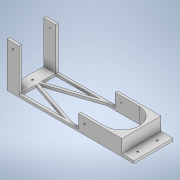
# Autodesk Inventor part: frame
Saved by Autodesk Inventor 2020 (Build 240168000, 168)
## iProperties
Created: 2020-02-29
Part Number: frame
Material: Типовые
Document SubType Name: Modeling
Designer: CSS38
Density: 1 g/cm^3
Appearance: По умолчанию
Author: CSS38
Autodesk Inventor part; units mm, degrees
ref_plane "YZ Plane" through (0, 0, 0) normal (1, 0, 0) x (0, 1, 0)
ref_plane "XZ Plane" through (0, 0, 0) normal (0, 1, 0) x (-1, 0, 0)
ref_plane "XY Plane" through (0, 0, 0) normal (0, 0, 1) x (1, 0, 0)
sketch "Эскиз1" plane through (0, 0, 0) normal (0, 1, 0) x (-1, 0, 0)
  line L0 (-52.75, 16.25) -> (52.75, 16.25)
  line L1 (52.75, 16.25) -> (52.75, -16.25)
  line L2 (52.75, -16.25) -> (-52.75, -16.25)
  line L3 (-52.75, -16.25) -> (-52.75, 16.25)
  line L4 (-52.75, 16.25) -> (52.75, -16.25) construction
  line L5 (52.75, 16.25) -> (-52.75, -16.25) construction
  line L6 (-42.75, -14.25) -> (0, -14.25)
  line L7 (42.75, -14.25) -> (42.75, -2.1082)
  line L8 (42.75, 14.25) -> (6.3246, 14.25)
  line L9 (-42.75, 14.25) -> (-42.75, -14.25)
  line L10 (52.75, -16.25) -> (36.5, 0) construction
  line L11 (36.5, 0) -> (52.75, 16.25) construction
  line L12 (47.75, -16.25) -> (47.75, 16.25) construction
  line L13 (0, -22.75) -> (0, 22.75) construction
  line L14 (0, -16.25) -> (0, -14.25) construction
  line L15 (0, 14.25) -> (0, 16.25) construction
  line L16 (0, -14.25) -> (42.75, 0)
  line L17 (42.75, 0) -> (0, 14.25)
  line L18 (42.75, -2.1082) -> (6.3246, -14.25)
  line L19 (42.75, 2.1082) -> (6.3246, 14.25)
  line L20 (42.75, -2.1082) -> (42.1175, -0.2108) construction
  line L21 (42.75, 2.1082) -> (42.1175, 0.2108) construction
  line L22 (42.75, -2.1082) -> (42.75, 2.1082) construction
  line L23 (42.75, 2.1082) -> (42.75, 14.25)
  line L24 (6.3246, -14.25) -> (42.75, -14.25)
  line L25 (0, -14.25) -> (6.3246, -14.25) construction
  line L26 (6.3246, 14.25) -> (0, 14.25) construction
  line L27 (0, 14.25) -> (-42.75, 14.25)
  point P0 (0, 0)
  point P1 (0, 0)
  dimension "d0" = 105.5
  dimension "d4" = 10
  dimension "d5" = 10
  dimension "d8" = 5
  dimension "d24" = 28.5
  dimension "d29" = 2
  constraints: 54 end point, 16 parallel, 14 perpendicular, 10 point on line, 5 equal length, 4 midpoint, 1 coincident, 1 horizontal
  measures "d0" distance of L1.end L2.end
  measures "d4" distance between parallel lines of L7 L1
  measures "d5" distance between parallel lines of L9 L3
  measures "d8" distance between parallel lines of L1 L12
  measures "d24" distance of L9.start L6.start
  measures "d29" distance of L14.start L6.end
extrude "Выдавливание1" add sketch "Эскиз1" along normal blind 2
sketch "Эскиз2" plane through (0, 0, 0) normal (0, 1, 0) x (-1, 0, 0)
  line L0 (-42.75, -16.25) -> (-42.75, 16.25)
  line L1 (52.75, 16.25) -> (-52.75, 16.25) projected
  line L2 (-52.75, 16.25) -> (-52.75, -16.25) projected
  line L3 (0, -14.25) -> (-42.75, -14.25) construction
  line L4 (-40.75, -14.25) -> (-40.75, 14.25) construction
  line L5 (6.3246, 14.25) -> (42.75, 14.25) construction
  line L6 (-40.75, -14.25) -> (-26.5, -14.25) construction
  line L7 (-6.75, -14.25) -> (-6.75, -16.25)
  line L8 (-52.75, -16.25) -> (52.75, -16.25) projected
  line L9 (-6.75, -16.25) -> (-42.75, -16.25)
  line L10 (-42.75, 16.25) -> (-6.75, 16.25)
  line L11 (-6.75, 14.25) -> (-26.5, 14.25)
  line L12 (-6.75, 14.25) -> (-6.75, 16.25)
  arc A0 (-26.5, 14.25) -> (-26.5, -14.25) centre (-26.5, 0) ccw
  line L13 (-26.5, -14.25) -> (-6.75, -14.25)
  line L14 (-26.5, 14.25) -> (-40.75, 14.25) construction
  line L15 (-42.75, -14.25) -> (-42.75, 14.25) projected
  point P0 (0, 0)
  point P1 (42.75, -14.25)
  point P2 (-42.75, -16.25)
  dimension "d13" = 2
  dimension "d14" = 34
  constraints: 20 end point, 7 point on line, 5 tangent, 4 collinear, 3 perpendicular, 3 vertical, 2 point on circle, 1 centre point
  measures "d13" distance between parallel lines of L0 L4
  measures "d14" distance of L4.start L7.start
extrude "Выдавливание2" add sketch "Эскиз2" along normal blind 13 contours L0 L1 L12 L11 A0 L13 L7 L8
sketch "Эскиз3" plane through (0, 2, 0) normal (0, 1, 0) x (1, 0, 0)
  line L0 (-42.75, 14.25) -> (-52.75, 14.25)
  line L1 (-52.75, 14.25) -> (-52.75, 16.25)
  line L2 (-52.75, 16.25) -> (-42.75, 16.25)
  line L3 (-42.75, 16.25) -> (-42.75, 14.25)
  line L4 (-52.75, 16.25) -> (-52.75, -16.25) construction
  line L5 (-52.75, -16.25) -> (-42.75, -16.25)
  line L6 (-42.75, -16.25) -> (-42.75, -14.25)
  line L7 (-42.75, -14.25) -> (-52.75, -14.25)
  line L8 (-52.75, -14.25) -> (-52.75, -16.25)
  point P0 (0, 0)
  point P1 (-42.75, 14.25)
  constraints: 16 end point, 4 parallel, 2 coincident, 2 horizontal, 2 perpendicular
extrude "Выдавливание3" add sketch "Эскиз3" along normal blind 35
sketch "Эскиз4" plane through (-52.75, 0, 16.25) normal (0, 0, 1) x (1, 0, 0)
  line L0 (10, 37) -> (0, 37) construction
  line L1 (0, 37) -> (10, 37) construction
  line L2 (10, 37) -> (10, 27) construction
  line L3 (10, 27) -> (0, 27) construction
  line L4 (0, 27) -> (0, 37) construction
  line L5 (105.5, 0) -> (0, 0) construction
  line L6 (0, 0) -> (0, 37) construction
  line L7 (10, 37) -> (10, 2) construction
  line L8 (10, 2) -> (59.5, 2) construction
  line L9 (59.5, 2) -> (59.5, 13) construction
  line L10 (59.5, 13) -> (95.5, 13) construction
  line L11 (95.5, 13) -> (95.5, 2) construction
  line L12 (95.5, 2) -> (105.5, 2) construction
  line L13 (105.5, 2) -> (105.5, 0) construction
  line L14 (10, 2) -> (10, 37) construction
  line L15 (0, 0) -> (0, 37) construction
  line L16 (10, 27) -> (0, 37) construction
  line L17 (10, 37) -> (0, 27) construction
  circle A0 centre (5, 32) radius 0.5
  line L18 (59.5, 13) -> (69.5, 13) construction
  line L19 (69.5, 13) -> (69.5, 3) construction
  line L20 (69.5, 3) -> (59.5, 3) construction
  line L21 (59.5, 3) -> (59.5, 13) construction
  line L22 (69.5, 13) -> (59.5, 3) construction
  line L23 (59.5, 2) -> (59.5, 13) construction
  line L24 (59.5, 13) -> (69.5, 3) construction
  circle A1 centre (64.5, 8) radius 0.5
  line L25 (0, 37) -> (10, 37) projected
  point P0 (52.75, 0)
  dimension "d19" = 1
  dimension "d20" = 10
  dimension "d21" = 1
  constraints: 24 end point, 5 perpendicular, 4 parallel, 2 centre point, 2 horizontal, 2 midpoint, 1 collinear
  measures "d19" diameter of A0
  measures "d20" distance of L19.end L20.end
  measures "d21" diameter of A1
hole "Отверстие1" at (-47.75, 32, 16.25) at (11.75, 8, 16.25) direction (0, 0, -1) diameter 1 depth 16.25 countersink diameter 1.5 countersink angle 90
mirror "Зеркальное отражение1" about plane through (0, 0, 0) normal (0, 0, 1) of "Отверстие1"
sketch "Эскиз5" plane through (0, 2, 0) normal (0, 1, 0) x (1, 0, 0)
  line L0 (-42.75, 2.1082) -> (-6.3246, 14.25) construction
  line L1 (-6.3246, 14.25) -> (-42.75, 14.25) construction
  line L2 (-42.75, 14.25) -> (-52.75, 14.25) construction
  line L3 (-52.75, -14.25) -> (-52.75, 14.25) construction
  line L4 (-52.75, -16.25) -> (-52.75, -14.25) construction
  line L5 (-42.75, -16.25) -> (-52.75, -16.25) construction
  line L6 (-42.75, -14.25) -> (-42.75, -16.25) construction
  line L7 (-42.75, -14.25) -> (-6.3246, -14.25) construction
  line L8 (-6.3246, -14.25) -> (-42.75, -2.1082) construction
  line L9 (-42.75, -2.1082) -> (-42.75, -14.25) construction
  line L10 (-42.75, 14.25) -> (-42.75, 2.1082) construction
  line L11 (-42.75, 16.25) -> (-42.75, 14.25) construction
  line L12 (-42.75, 16.25) -> (6.75, 16.25) construction
  line L13 (6.75, 16.25) -> (42.75, 16.25) construction
  line L14 (42.75, 16.25) -> (52.75, 16.25) construction
  line L15 (52.75, 16.25) -> (52.75, -16.25) construction
  line L16 (52.75, -16.25) -> (42.75, -16.25) construction
  line L17 (42.75, 16.25) -> (42.75, -16.25) construction
  line L18 (-52.75, 14.25) -> (-52.75, 16.25) construction
  line L19 (-52.75, 16.25) -> (-42.75, 16.25) construction
  line L20 (-52.75, -14.25) -> (-42.75, -14.25) construction
  line L21 (6.75, -16.25) -> (-42.75, -16.25) construction
  line L22 (42.75, -16.25) -> (6.75, -16.25) construction
  line L23 (6.75, 14.25) -> (6.75, 16.25) construction
  line L24 (6.75, 14.25) -> (0, 14.25) construction
  line L25 (0, 14.25) -> (-42.75, 0) construction
  line L26 (-42.75, 0) -> (0, -14.25) construction
  line L27 (0, -14.25) -> (6.75, -14.25) construction
  line L28 (6.75, -14.25) -> (26.5, -14.25) construction
  arc A0 (26.5, -14.25) -> (26.5, 14.25) centre (26.5, 0) ccw construction
  line L29 (26.5, 14.25) -> (6.75, 14.25) construction
  line L30 (6.75, -16.25) -> (6.75, -14.25) construction
  line L31 (-6.3246, -14.25) -> (-42.75, -14.25) construction
  line L32 (-52.75, 14.25) -> (-42.75, -14.25) construction
  line L33 (-42.75, 14.25) -> (-52.75, -14.25) construction
  line L34 (42.75, 16.25) -> (52.75, 0) construction
  line L35 (52.75, -16.25) -> (52.75, 16.25) construction
  line L36 (52.75, 0) -> (42.75, -16.25) construction
  line L37 (-52.75, -16.25) -> (52.75, -16.25) construction
  line L38 (52.75, -16.25) -> (42.75, 0) construction
  line L39 (52.75, 16.25) -> (-52.75, 16.25) construction
  line L40 (42.75, 0) -> (52.75, 16.25) construction
  circle A1 centre (-47.75, 0) radius 0.5
  circle A2 centre (47.75, 8.125) radius 0.5
  circle A3 centre (47.75, -8.125) radius 0.5
  point P0 (0, 0)
  dimension "d37" = 1
  constraints: 12 end point, 5 midpoint, 3 centre point, 2 equal radius, 1 parallel
  measures "d37" diameter of A1
hole "Отверстие2" at (-47.75, 2, 0) at (47.75, 2, -8.125) at (47.75, 2, 8.125) direction (0, -1, 0) diameter 1 end through all countersink diameter 1.5 countersink angle 90
